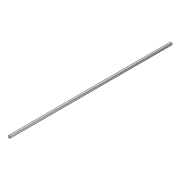
# Autodesk Inventor part: FE-00004-05
Saved by Autodesk Inventor 2012 (Build 160160000, 160)
## iProperties
Created: 2008-05-29
Part Number: FE-00004-05
Document SubType Name: Modeling
Designer: narosenberg
Density: 1 g/cm^3
Description: Support, Window
Mass: 294.967 g
Surface Area: 1977.42 cm^2
Volume: 294.967 cm^3
Material: Default
Author: narosenberg
Autodesk Inventor part; units mm, degrees
ref_plane "YZ Plane" through (0, 0, 0) normal (1, 0, 0) x (0, 1, 0)
ref_plane "XZ Plane" through (0, 0, 0) normal (0, 1, 0) x (-1, 0, 0)
ref_plane "XY Plane" through (0, 0, 0) normal (0, 0, 1) x (1, 0, 0)
sketch "Sketch1" plane through (0, 0, 0) normal (0, 0, 1) x (1, 0, 0)
  line L0 (-16.8285, 19.5793) -> (2.2215, 19.5793)
  line L1 (2.2215, 19.5793) -> (2.2215, 0.5293)
  line L2 (2.2215, 0.5293) -> (-16.8285, 0.5293)
  line L3 (-16.8285, 0.5293) -> (-16.8285, 19.5793)
  line L4 (-16.8285, 16.4043) -> (-0.9535, 16.4043)
  line L5 (-0.9535, 16.4043) -> (-0.9535, 3.7043)
  line L6 (-0.9535, 3.7043) -> (-16.8285, 3.7043)
  line L7 (-16.8285, 3.7043) -> (-16.8285, 16.4043)
  dimension "d0" = 19.05
  dimension "d1" = 19.05
  dimension "d2" = 3.175
  dimension "d3" = 3.175
  dimension "d4" = 3.175
  constraints: 16 end point, 4 parallel, 2 horizontal, 2 perpendicular, 1 point on line
  measures "d0" distance of L0.start L0.end
  measures "d1" distance of L0.end L1.end
  measures "d2" distance between parallel lines of L0 L4
  measures "d3" distance between parallel lines of L1 L5
  measures "d4" distance between parallel lines of L2 L6
extrude "Extrusion1" add sketch "Sketch1" along normal blind 1701.8 contours L0 L1 L2 L3 L6 L5 L4
body "Solid1"
